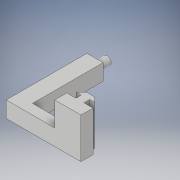
# Autodesk Inventor part: Grab Rail v2.5 - Left
Saved by Autodesk Inventor 2018 (Build 220112000, 112)
## iProperties
Created: 2019-12-12
Part Number: Grab Rail v2.5 - Left
Material: Generic
Document SubType Name: Modeling
Designer: AOFUser
Density: 1 g/cm^3
Appearance: Default
Author: AOFUser
Autodesk Inventor part; units mm, degrees
ref_plane "YZ Plane" through (0, 0, 0) normal (1, 0, 0) x (0, 1, 0)
ref_plane "XZ Plane" through (0, 0, 0) normal (0, 1, 0) x (-1, 0, 0)
ref_plane "XY Plane" through (0, 0, 0) normal (0, 0, 1) x (1, 0, 0)
sketch "Sketch1" plane through (0, 0, 0) normal (0, 1, 0) x (-1, 0, 0)
  line L0 (0, 0) -> (16.51, 0)
  line L1 (16.51, 0) -> (16.51, 7.62)
  line L2 (16.51, 7.62) -> (0, 7.62)
  line L3 (0, 7.62) -> (0, 0)
  line L4 (16.51, 0) -> (10.795, 0)
  line L5 (10.795, 0) -> (10.795, -6.604)
  line L6 (10.795, -6.604) -> (5.715, -6.604)
  line L7 (5.715, -6.604) -> (5.715, 0)
  line L8 (5.715, -6.604) -> (5.715, -3.556)
  line L9 (5.715, -3.556) -> (2.667, -3.556)
  line L10 (2.667, -3.556) -> (5.715, -6.604)
  line L11 (10.795, -3.302) -> (13.843, -3.302)
  line L12 (13.843, -3.302) -> (10.795, -6.604)
  dimension "d0" = 16.51
  dimension "d1" = 7.62
  dimension "d2" = 5.715
  dimension "d3" = 6.604
  dimension "d4" = 5.08
  dimension "d5" = 3.048
  dimension "d6" = 3.048
  dimension "d7" = 3.048
  constraints: 26 end point, 5 perpendicular, 3 point on line, 2 horizontal, 2 parallel, 1 midpoint
  measures "d0" distance of L2.end L1.end
  measures "d1" distance of L1.end L0.end
  measures "d2" distance of L0.end L4.end
  measures "d3" distance of L4.end L5.end
  measures "d4" distance of L5.end L6.end
  measures "d5" distance of L6.end L8.end
  measures "d6" distance of L8.end L9.end
  measures "d7" distance of L11.start L11.end
extrude "Extrusion1" add sketch "Sketch1" along normal blind 25.4
sketch "Sketch3" plane through (-16.51, 0, 0) normal (-1, 0, 0) x (0, 0, 1)
  line L0 (0, 0) -> (7.62, 0) projected
  line L1 (7.62, 0) -> (1.27, 0)
  line L2 (1.27, 0) -> (1.27, 10.16)
  line L3 (1.27, 10.16) -> (7.62, 10.16)
  line L4 (7.62, 10.16) -> (7.62, 0)
  dimension "d10" = 6.35
  dimension "d11" = 10.16
  constraints: 8 end point, 2 parallel, 1 horizontal, 1 perpendicular
  measures "d10" distance of L2.end L3.end
  measures "d11" distance of L1.end L2.end
extrude "Extrusion2" add sketch "Sketch3" along normal blind 30.48
sketch "Sketch4" plane through (-16.51, 0, 1.27) normal (0, 0, -1) x (-1, 0, 0)
  line L0 (30.48, 10.16) -> (30.48, 0) projected
  line L1 (30.48, 10.16) -> (20.32, 10.16)
  line L2 (20.32, 10.16) -> (20.32, 0)
  line L3 (20.32, 0) -> (30.48, 0)
  line L4 (30.48, 0) -> (30.48, 10.16)
  point P0 (-16.51, 0)
  dimension "d14" = 10.16
  dimension "d15" = 10.16
  constraints: 8 end point, 2 parallel, 1 horizontal, 1 perpendicular
  measures "d14" distance of L3.end L2.end
  measures "d15" distance of L2.end L1.end
extrude "Extrusion3" add sketch "Sketch4" along normal blind 44.45
sketch "Sketch5" plane through (-16.51, 0, -43.18) normal (0, 0, -1) x (-1, 0, 0)
  line L0 (30.48, 0) -> (30.48, 10.16) projected
  line L1 (30.48, 5.08) -> (25.4, 5.08)
  circle A0 centre (25.4, 5.08) radius 2.54
  point P0 (-16.51, 0)
  dimension "d18" = 5.08
  dimension "d19" = 5.08
  constraints: 2 end point, 1 centre point, 1 coincident, 1 horizontal, 1 midpoint
  measures "d18" distance of L1.start L1.end
  measures "d19" diameter of A0
extrude "Extrusion4" add sketch "Sketch5" along normal blind 7.62
sketch "Sketch6" plane through (-41.91, 5.08, -50.8) normal (0, 0, -1) x (-1, 0, 0)
  circle A0 centre (0, 0) radius 2.54 projected
  line L0 (2.54, 0) -> (0, 0)
  point P0 (-41.91, -5.08)
  constraints: 2 end point, 1 horizontal, 1 horizontal alignment, 1 other
hole "Hole1" at (-41.91, 5.08, -50.8) direction (0, 0, 1) diameter 2.794 depth 16.002 tip angle 118
body "Solid1"
